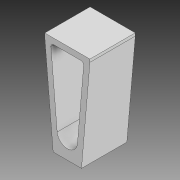
# Autodesk Inventor part: MainBracketY
Saved by Autodesk Inventor 2020 (Build 240168000, 168)
## iProperties
Created: 2021-01-14
Part Number: MainBracketY
Material: Generic
Document SubType Name: Modeling
Designer: DDeGo
Density: 1 g/cm^3
Appearance: Default
Author: DDeGo
Autodesk Inventor part; units mm, degrees
ref_plane "YZ Plane" through (0, 0, 0) normal (1, 0, 0) x (0, 1, 0)
ref_plane "XZ Plane" through (0, 0, 0) normal (0, 1, 0) x (-1, 0, 0)
ref_plane "XY Plane" through (0, 0, 0) normal (0, 0, 1) x (1, 0, 0)
sketch "Sketch1" plane through (0, 0, 0) normal (0, 0, 1) x (1, 0, 0)
  line L0 (0, 0) -> (0, 17.4353) construction
  line L1 (0, 17.4353) -> (-3.9816, 17.4353)
  line L2 (-3.9816, 17.4353) -> (-3.9816, 16.9353)
  line L3 (-3.9816, 16.9353) -> (-2.5, 0)
  line L4 (-2.5, 0) -> (0, 0)
  line L5 (0, 17.4353) -> (3.9816, 17.4353)
  line L6 (3.9816, 17.4353) -> (3.9816, 16.9353)
  line L7 (3.9816, 16.9353) -> (2.5, 0)
  line L8 (2.5, 0) -> (0, 0)
  line L9 (-2.3884, 16.4353) -> (1.8987, 16.4353)
  line L10 (1.8987, 16.4353) -> (2.3884, 16.4353)
  line L11 (2.8865, 15.8917) -> (1.794, 3.4039)
  line L12 (-1.794, 3.4039) -> (-2.8865, 15.8917)
  arc A0 (-2.3884, 16.4353) -> (-2.8865, 15.8917) centre (-2.3884, 15.9353) ccw
  arc A1 (2.8865, 15.8917) -> (2.3884, 16.4353) centre (2.3884, 15.9353) ccw
  arc A2 (-1.794, 3.4039) -> (1.794, 3.4039) centre (0, 3.5609) ccw
  point P0 (-2.9341, 16.4353)
  point P1 (2.9341, 16.4353)
  point P2 (0, -17.1014)
  point P3 (1.8884, 16.4353)
  dimension "d1" = 5
  dimension "d2" = 0.5
  dimension "d3" = 17
  dimension "d4" = 1
  dimension "d7" = 0.5
  dimension "d8" = 5
  constraints: 26 end point, 6 point on circle, 6 point on line, 6 tangent, 3 centre point, 3 symmetric about line, 2 perpendicular, 1 equal radius, 1 parallel, 1 vertical, 3 other
  measures "d1" angle of L0 L3
  measures "d2" distance of L1.end L2.end
  measures "d3" distance of L2.end L3.end
  measures "d4" distance between parallel lines of L1 L9
  measures "d7" radius of A0
  measures "d8" distance of L7.end L3.end
extrude "Extrusion1" add sketch "Sketch1" along normal blind 8
body "Solid1"
